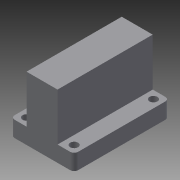
# Autodesk Inventor part: Near Gantry Bracket
Saved by Autodesk Inventor 2015 (Build 190159000, 159)
## iProperties
Created: 2016-04-12
Part Number: Near Gantry Bracket
Material: Generic
Document SubType Name: Modeling
Designer: rubenjm
Density: 1 g/cm^3
Appearance: Default
Author: rubenjm
Autodesk Inventor part; units mm, degrees
ref_plane "YZ Plane" through (0, 0, 0) normal (1, 0, 0) x (0, 1, 0)
ref_plane "XZ Plane" through (0, 0, 0) normal (0, 1, 0) x (-1, 0, 0)
ref_plane "XY Plane" through (0, 0, 0) normal (0, 0, 1) x (1, 0, 0)
sketch "Sketch1" plane through (0, 0, 0) normal (0, 1, 0) x (-1, 0, 0)
  line L0 (3.175, 0) -> (47.625, 0)
  line L1 (50.8, -3.175) -> (50.8, -73.025)
  line L2 (47.625, -76.2) -> (3.175, -76.2)
  line L3 (0, -73.025) -> (0, -3.175)
  arc A0 (50.8, -3.175) -> (47.625, 0) centre (47.625, -3.175) ccw
  arc A1 (3.175, 0) -> (0, -3.175) centre (3.175, -3.175) ccw
  arc A2 (0, -73.025) -> (3.175, -76.2) centre (3.175, -73.025) ccw
  arc A3 (47.625, -76.2) -> (50.8, -73.025) centre (47.625, -73.025) ccw
  point P0 (0, 0)
  point P1 (50.8, -76.2)
  point P2 (50.8, 0)
  point P3 (0, -76.2)
  dimension "d0" = 50.8
  dimension "d1" = 76.2
  dimension "d4" = 3.175
  constraints: 8 end point, 8 point on circle, 8 point on line, 8 tangent, 4 centre point, 3 equal radius, 2 parallel, 1 horizontal, 1 perpendicular
  measures "d0" distance of point (50.8, -76.2) point (0, -76.2)
  measures "d1" distance of point (50.8, 0) point (50.8, -76.2)
  measures "d4" radius of A0
extrude "Extrusion1" add sketch "Sketch1" along normal blind 12.7
sketch "Sketch2" plane through (0, 12.7, 0) normal (0, 1, 0) x (1, 0, 0)
  line L0 (0, 0) -> (-6.35, 0) construction
  line L1 (-6.35, 0) -> (-6.35, 6.35) construction
  line L2 (-6.35, 6.35) -> (0, 6.35) construction
  line L3 (0, 6.35) -> (0, 0) construction
  circle A0 centre (-6.35, 6.35) radius 3.175
  line L4 (0, 3.175) -> (0, 73.025) construction
  line L5 (0, 38.1) -> (-50.8802, 38.1) construction
  line L6 (-50.8802, 38.1) -> (-25.4, 76.2) construction
  line L7 (-3.175, 76.2) -> (-47.625, 76.2) construction
  line L8 (-25.4, 76.2) -> (-25.4, 0) construction
  line L9 (-47.625, 0) -> (-3.175, 0) construction
  circle A1 centre (-6.35, 69.85) radius 3.175
  circle A2 centre (-44.45, 6.35) radius 3.175
  circle A3 centre (-44.45, 69.85) radius 3.175
  dimension "d5" = 6.35
  dimension "d6" = 6.35
  dimension "d7" = 6.35
  constraints: 14 end point, 4 centre point, 3 midpoint, 3 symmetric about line, 2 horizontal, 2 parallel, 1 coincident, 1 perpendicular, 3 other
  measures "d5" distance of L1.end L2.end
  measures "d6" distance of L0.end L1.end
  measures "d7" diameter of A0
extrude "Extrusion2" cut sketch "Sketch2" against normal through all
sketch "Sketch3" plane through (0, 12.7, 0) normal (0, 1, 0) x (1, 0, 0)
  line L0 (0, 0) -> (-12.7, 0) construction
  line L1 (0, 0) -> (12.7, 0) construction
  line L2 (-47.625, 0) -> (-3.175, 0) construction
  line L3 (-25.4, 0) -> (-25.4, 76.2) construction
  line L4 (-3.175, 76.2) -> (-47.625, 76.2) construction
  line L5 (-50.8, 0) -> (-38.1, 0) construction
  line L6 (-38.1, 0) -> (-13.2855, 0)
  line L7 (-13.2855, 0) -> (-13.2855, 76.2)
  line L8 (-13.2855, 76.2) -> (-38.1, 76.2)
  line L9 (-38.1, 76.2) -> (-38.1, 0)
  dimension "d14" = 12.7
  dimension "d15" = 180
  constraints: 16 end point, 3 horizontal, 2 midpoint, 2 parallel, 2 symmetric about line, 1 collinear, 1 perpendicular, 1 point on line
  measures "d14" distance of L0.start L0.end
  measures "d15" angle of L0 L1
extrude "Extrusion3" add sketch "Sketch3" along normal blind 38.1
sketch "Sketch4" plane through (0, 0, 0) normal (0, -1, 0) x (1, 0, 0)
  line L0 (0, 0) -> (-12.7, 0) construction
  line L1 (-12.7, 0) -> (-12.7, -12.7) construction
  line L2 (-12.7, -12.7) -> (0, -12.7) construction
  line L3 (0, -12.7) -> (0, 0) construction
  line L4 (-50.8, -76.2) -> (-38.1, -76.2) construction
  line L5 (-38.1, -76.2) -> (-38.1, -63.5) construction
  line L6 (-38.1, -63.5) -> (-50.8, -63.5) construction
  line L7 (-50.8, -63.5) -> (-50.8, -76.2) construction
  line L8 (-12.7, -12.7) -> (-38.1, -12.7)
  line L9 (-38.1, -12.7) -> (-38.1, -63.5)
  line L10 (-38.1, -63.5) -> (-12.7, -63.5)
  line L11 (-12.7, -63.5) -> (-12.7, -12.7)
  dimension "d18" = 12.7
  dimension "d19" = 12.7
  dimension "d20" = 12.7
  dimension "d21" = 12.7
  constraints: 24 end point, 6 parallel, 3 horizontal, 3 perpendicular
  measures "d18" distance of L2.end L1.end
  measures "d19" distance of L1.end L0.end
  measures "d20" distance of L6.end L5.end
  measures "d21" distance of L5.end L4.end
extrude "Extrusion4" cut sketch "Sketch4" against normal blind 6.35
body "Solid1"
